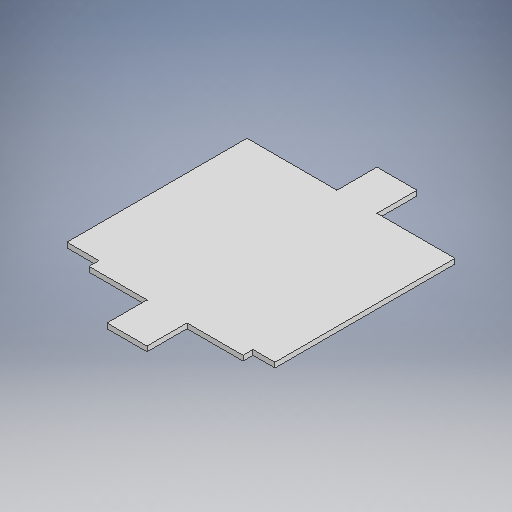
# Autodesk Inventor part: imu_seat
Saved by Autodesk Inventor 2025.2 (Build 292293000, 293)
## iProperties
Created: 2025-02-02
Part Number: imu_seat
Material: 일반
Document SubType Name: Modeling
Designer: jbhma
Density: 1 g/cm^3
Appearance: 기본값
Author: jbhma
Autodesk Inventor part; units mm, degrees
ref_plane "YZ Plane" through (0, 0, 0) normal (1, 0, 0) x (0, 1, 0)
ref_plane "XZ Plane" through (0, 0, 0) normal (0, 1, 0) x (-1, 0, 0)
ref_plane "XY Plane" through (0, 0, 0) normal (0, 0, 1) x (1, 0, 0)
sketch "스케치1" plane through (0, 0, 0) normal (0, 1, 0) x (-1, 0, 0)
  line L0 (-69.1144, 67.9118) -> (34.8856, 67.9118)
  line L1 (34.8856, 67.9118) -> (34.8856, -22.0882)
  line L2 (34.8856, -22.0882) -> (-69.1144, -22.0882)
  line L3 (-69.1144, -22.0882) -> (-69.1144, 67.9118)
  line L4 (-10.1144, -22.0882) -> (-30.1144, -22.0882)
  line L5 (-30.1144, -22.0882) -> (-30.1144, -42.0882)
  line L6 (-30.1144, -42.0882) -> (-10.1144, -42.0882)
  line L7 (-10.1144, -42.0882) -> (-10.1144, -22.0882)
  line L8 (18.8856, 67.9118) -> (-58.1144, 67.9118)
  line L9 (-58.1144, 67.9118) -> (-58.1144, 72.9118)
  line L10 (-58.1144, 72.9118) -> (18.8856, 72.9118)
  line L11 (18.8856, 72.9118) -> (18.8856, 67.9118)
  line L12 (-30.1144, 72.9118) -> (-10.1144, 72.9118)
  line L13 (-10.1144, 72.9118) -> (-10.1144, 92.9118)
  line L14 (-10.1144, 92.9118) -> (-30.1144, 92.9118)
  line L15 (-30.1144, 92.9118) -> (-30.1144, 72.9118)
  point P0 (0, 0)
  point P1 (-20.1144, -42.0882)
  point P2 (-58.1144, 70.4118)
  point P3 (18.8856, 70.4118)
  dimension "d10" = 90
  dimension "d11" = 104
  dimension "d12" = 39
  dimension "d13" = 59
  dimension "d14" = 20
  dimension "d15" = 5
  dimension "d16" = 11
  dimension "d17" = 16
  dimension "d18" = 39
  dimension "d19" = 59
  dimension "d20" = 20
  constraints: 32 end point, 8 parallel, 4 horizontal, 4 perpendicular, 3 midpoint, 3 point on line
  measures "d10" distance between parallel lines of L2 L0
  measures "d11" distance between parallel lines of L3 L1
  measures "d12" distance between parallel lines of L3 L5
  measures "d13" distance between parallel lines of L3 L7
  measures "d14" distance from line of point (-20.114, -42.088) L2
  measures "d15" distance between parallel lines of L0 L10
  measures "d16" distance from line of L3 point (-58.114, 70.412)
  measures "d17" distance from line of L1 point (18.886, 70.412)
  measures "d18" distance between parallel lines of L3 L15
  measures "d19" distance between parallel lines of L3 L13
  measures "d20" distance between parallel lines of L10 L14
extrude "돌출1" add sketch "스케치1" along normal blind 2.5
